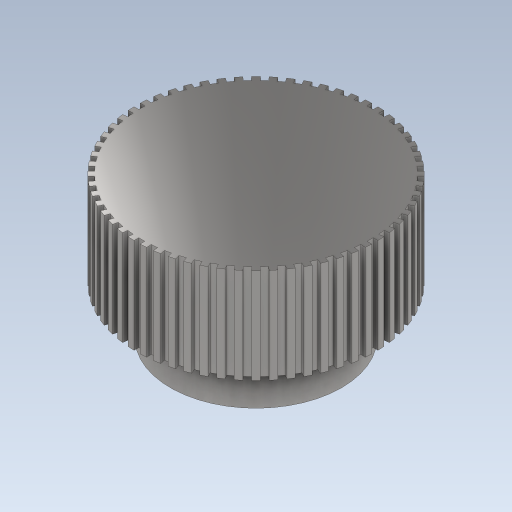
# Autodesk Inventor part: Pump-Motor-CW-Rotation:Cover 103
Saved by Autodesk Inventor 2024.2 (Build 282272000, 272)
## iProperties
Created: 2025-06-16
Material: Steel
Document SubType Name: Modeling
Density: 7.85 g/cm^3
Appearance: Semi-Polished
Designer: cw
Author: cw
Autodesk Inventor part; units mm, degrees
ref_plane "YZ Plane" through (0, 0, 0) normal (1, 0, 0) x (0, 1, 0)
ref_plane "XZ Plane" through (0, 0, 0) normal (0, 1, 0) x (-1, 0, 0)
ref_plane "XY Plane" through (0, 0, 0) normal (0, 0, 1) x (1, 0, 0)
sketch "Sketch1" plane through (0, 0, 0) normal (0, 1, 0) x (-1, 0, 0)
  line L0 (0, 0) -> (-12.5, 0)
  line L1 (-12.5, 0) -> (-12.5, -10)
  line L2 (-12.5, -10) -> (-9, -10)
  line L3 (-9, -10) -> (-9, -15)
  line L4 (-9, -15) -> (0, -15)
  line L5 (0, -15) -> (0, 0)
  line L6 (0, -7) -> (-6, -7)
  line L7 (-6, -7) -> (-6, -3.4674)
  arc A0 (0, -2) -> (-6, -3.4674) centre (0, -15) ccw
  dimension "d3" = 25
  dimension "d4" = 18
  dimension "d5" = 10
  dimension "d6" = 5
  dimension "d22" = 12
  dimension "d23" = 8
  dimension "d24" = 13
  constraints: 16 end point, 7 perpendicular, 2 point on circle, 2 point on line, 1 centre point, 1 horizontal
  measures "d3" diameter of L1 L5
  measures "d4" diameter of L3 L5
  measures "d5" distance of L0.end L1.end
  measures "d6" distance between parallel lines of L4 L2
  measures "d22" diameter of L7 L5
  measures "d23" distance between parallel lines of L6 L4
  measures "d24" distance from line of L4 A0.start
revolve "Revolution1" add sketch "Sketch1" angle 360 about axis through (0, 0, -15) along (0, 0, 1) contours L5 A0 L7 L6 L4 L3 L2 L1 L0
sketch "Sketch2" plane through (0, 0, -15) normal (0, 0, -1) x (-1, 0, 0)
  point P0 (0, 0)
hole "Hole1" at (0, 0, -15) direction (0, 0, 1) diameter 10.106 depth 8 thread size "M12x1.75" class "6H" standard "ISO Metric profile"
sketch "Sketch3" plane through (0, 0, 0) normal (0, 0, 1) x (1, 0, 0)
  line L0 (0, 0) -> (-0.3272, -12.4957)
  circle A0 centre (0, 0) radius 12.5 projected
  line L1 (0, 0) -> (0.3272, -12.4957)
  arc A1 (-0.3141, -11.9959) -> (0.3141, -11.9959) centre (0, 0) ccw
  dimension "d15" = 3
  dimension "d16" = 12
  constraints: 4 end point, 4 point on circle, 2 point on line, 1 centre point, 1 coincident, 1 horizontal alignment
  measures "d15" angle of L1 L0
  measures "d16" radius of A1
extrude "Extrusion1" cut sketch "Sketch3" against normal through all contours A1 L1 A0 L0
pattern_circular "Circular Pattern1" count 60 over 360 about axis through (0, 0, -10) along (0, 0, 1) of "Extrusion1"
fillet "Fillet1" radius 2 1 edges at (-6, 0, -3.4674)
body "Solid1"
